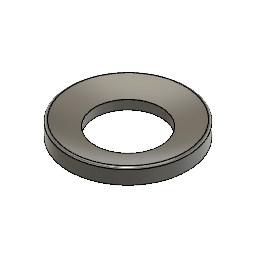
Ring (Autodesk Fusion 360 design; units mm, degrees)
Autodesk Fusion 360 part; units mm, degrees
sketch "Sketch1" plane through (0, 0, 0) normal (0, 1, 0) x (1, 0, 0)
  circle A0 centre (0, 0) radius 1.625
  dimension "d1" = 3.25
  measures "d1" diameter of A0
extrude "Extrude1" add sketch "Sketch1" along normal blind 0.44
ref_plane "WorkPlane1" through (-0.3108, 0.0895, 1.595) normal (-0.191241, 0, 0.981543) x (-0.981543, 0, -0.191241)
ref_plane "WorkPlane2" through (0, 0.0895, 0) normal (-0.191241, 0, 0.981543) x (-0.981543, 0, -0.191241)
sketch "Sketch2" plane through (0, 0.0895, 0) normal (-0.191241, 0, 0.981543) x (-0.981543, 0, -0.191241)
  arc A0 (1.625, -0.3505) -> (-1.625, -0.3505) centre (0, -5.0791) ccw
  line L0 (-1.625, -0.3505) -> (1.625, -0.3505)
  line L1 (0, -3.3) -> (0, -2.7)
  line L2 (1.625, -0.3505) -> (-1.625, -0.3505)
  line L3 (0, -0.0791) -> (0, -0.3505)
  dimension "d6" = 5
  measures "d6" radius of A0
revolve "Revolve1" cut sketch "Sketch2" angle 360 about axis through (0, 1.75, 0) along (0, 1, 0) contours A0 L0 L2 L3 picked at (-0.1835, -0.1797)
sketch "Sketch3" plane through (0, 0, 0) normal (0, -1, 0) x (1, 0, 0)
  circle A0 centre (0, 0) radius 1.625
  circle A1 centre (0, 0) radius 0.9
  dimension "d8" = 1.8
  measures "d8" diameter of A1
extrude "Extrude2" cut sketch "Sketch3" against normal through all contours A1
fillet "Fillet1" radius 0.05 1 edges at (-1.515, 0.44, 0.5876)
